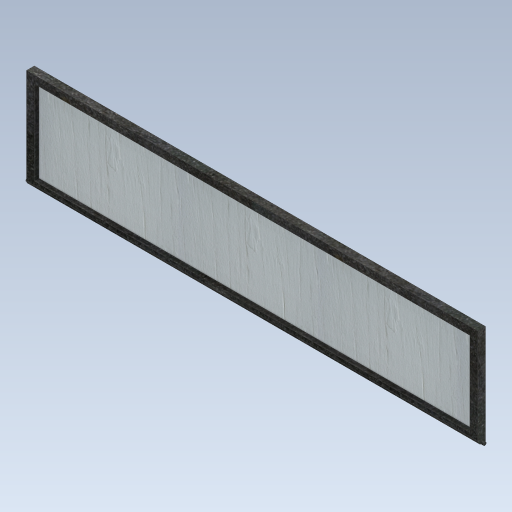
# Autodesk Inventor part: puerta
Saved by Autodesk Inventor 2023 (Build 270158000, 158)
## iProperties
Created: 2023-03-08
Part Number: puerta
Material: Steel
Document SubType Name: Modeling
Designer: santi
Density: 7.85 g/cm^3
Appearance: Plate
Author: santi
Autodesk Inventor part; units mm, degrees
ref_plane "YZ Plane" through (0, 0, 0) normal (1, 0, 0) x (0, 1, 0)
ref_plane "XZ Plane" through (0, 0, 0) normal (0, 1, 0) x (-1, 0, 0)
ref_plane "XY Plane" through (0, 0, 0) normal (0, 0, 1) x (1, 0, 0)
sketch "Sketch1" plane through (0, 0, 0) normal (0, 0, 1) x (1, 0, 0)
  line L0 (0, 0) -> (290, 0)
  line L1 (290, 0) -> (290, 64.12)
  line L2 (290, 64.12) -> (0, 64.12)
  line L3 (0, 64.12) -> (0, 0)
  line L4 (5, 59.12) -> (285, 59.12)
  line L5 (285, 59.12) -> (285, 5)
  line L6 (285, 5) -> (5, 5)
  line L7 (5, 5) -> (5, 59.12)
  dimension "d0" = 290
  dimension "d1" = 64.12
  dimension "d2" = 5
  constraints: 16 end point, 4 parallel, 2 perpendicular, 1 horizontal, 3 other
  measures "d0" distance of L2.end L1.end
  measures "d1" distance of L1.end L0.end
  measures "d2" distance between parallel lines of L2 L4
extrude "Extrusion1" add sketch "Sketch1" along normal blind 5
sketch "Sketch2" plane through (5, 5, 0) normal (1, 0, 0) x (0, 0, -1)
  line L0 (0, 54.12) -> (0, 0) projected
  line L1 (0, 54.12) -> (-5, 54.12) projected
  line L2 (0, 0) -> (-2, 0)
  line L3 (-2, 0) -> (-2, 54.12)
  line L4 (-2, 54.12) -> (0, 54.12)
  line L5 (0, 54.12) -> (0, 0)
  point P0 (0, -5)
  dimension "d5" = 2
  constraints: 8 end point, 2 parallel, 1 horizontal, 1 perpendicular, 1 point on line
  measures "d5" distance of L3.end L4.end
extrude "Extrusion2" add sketch "Sketch2" along normal up to surface (280 mm away)
sketch "Sketch3" plane through (0, 0, 0) normal (-1, 0, 0) x (0, 0, 1)
  circle A0 centre (2.5, 1) radius 1
  line L0 (5, 64.12) -> (5, 0) construction
  line L1 (0, 0) -> (5, 0) construction
  point P0 (2.5, 0)
  dimension "d8" = 2
  constraints: 1 centre point, 1 midpoint, 1 tangent, 1 vertical alignment
  measures "d8" diameter of A0
extrude "Extrusion3" add sketch "Sketch3" along normal blind 2 and the other way blind 2
ref_plane "Work Plane1" through (145, 0, 0) normal (1, 0, 0) x (0, 0, -1)
mirror "Mirror1" about plane through (145, 0, 0) normal (1, 0, 0) of "Extrusion3"
fillet "Fillet1" radius 2.7 1 edges at (145, 0, 5)
body "Solid1"
